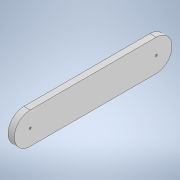
# Autodesk Inventor part: first_arm
Saved by Autodesk Inventor 2022 (Build 260153000, 153)
## iProperties
Created: 2022-02-25
Part Number: first_arm
Material: Generic
Document SubType Name: Modeling
Designer: Dan
Density: 1 g/cm^3
Appearance: Default
Author: Dan
Autodesk Inventor part; units mm, degrees
ref_plane "YZ Plane" through (0, 0, 0) normal (1, 0, 0) x (0, 1, 0)
ref_plane "XZ Plane" through (0, 0, 0) normal (0, 1, 0) x (-1, 0, 0)
ref_plane "XY Plane" through (0, 0, 0) normal (0, 0, 1) x (1, 0, 0)
sketch "Sketch1" plane through (0, 0, 0) normal (1, 0, 0) x (0, 1, 0)
  arc A0 (25, 0) -> (-25, 0) centre (0, 0) ccw
  line L0 (-25, 0) -> (-25, -200)
  line L1 (25, 0) -> (25, -200)
  arc A1 (-25, -200) -> (25, -200) centre (0, -200) ccw
  dimension "d0" = 50
  dimension "d2" = 200
  constraints: 4 end point, 4 point on circle, 2 centre point, 2 tangent, 2 vertical, 1 coincident, 1 equal radius
  measures "d0" diameter of A0
  measures "d2" distance of L0.start L0.end
extrude "Extrusion1" add sketch "Sketch1" along normal blind 10
sketch "Sketch2" plane through (10, 0, 0) normal (1, 0, 0) x (0, 0, -1)
  arc A0 (200, -25) -> (200, 25) centre (200, 0) ccw projected
  point P0 (0, 0)
  point P1 (0, 0)
  point P2 (200, 0)
  constraints: 2 coincident
hole "Hole1" at (10, 0, 0) at (10, 0, -200) direction (-1, 0, 0) diameter 3 end through all
body "Solid1"
